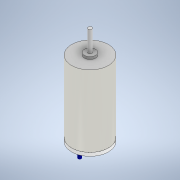
# Autodesk Inventor part: motor_noname
Saved by Autodesk Inventor 2021 (Build 250183000, 183)
## iProperties
Created: 2022-02-27
Part Number: motor_noname
Material: Generic
Document SubType Name: Modeling
Designer: ermoz
Density: 1 g/cm^3
Appearance: Default
Author: ermoz
Autodesk Inventor part; units mm, degrees
ref_plane "YZ Plane" through (0, 0, 0) normal (1, 0, 0) x (0, 1, 0)
ref_plane "XZ Plane" through (0, 0, 0) normal (0, 1, 0) x (-1, 0, 0)
ref_plane "XY Plane" through (0, 0, 0) normal (0, 0, 1) x (1, 0, 0)
sketch "Sketch1" plane through (0, 0, 0) normal (0, 1, 0) x (-1, 0, 0)
  circle A0 centre (0, 0) radius 4
  dimension "d0" = 8
  constraints: 1 centre point, 1 coincident
  measures "d0" diameter of A0
extrude "Extrusion1" add sketch "Sketch1" along normal blind 15.6
sketch "Sketch2" plane through (0, 15.6, 0) normal (0, 1, 0) x (1, 0, 0)
  circle A0 centre (0, 0) radius 4 projected
  circle A1 centre (0, 0) radius 1.2
  dimension "d3" = 2.4
  constraints: 1 centre point, 1 coincident
  measures "d3" diameter of A1
extrude "Extrusion2" add sketch "Sketch2" along normal blind 0.5 contours A1
sketch "Sketch3" plane through (0, 0, 0) normal (0, -1, 0) x (1, 0, 0)
  circle A0 centre (0, 0) radius 1.2 projected
  circle A1 centre (0, 0) radius 4
  constraints: 1 centre point, 1 coincident
extrude "Extrusion3" add sketch "Sketch3" along normal blind 0.75 separate body contours A0 | A1
sketch "Sketch4" plane through (0, 16.1, 0) normal (0, 1, 0) x (1, 0, 0)
  circle A0 centre (0, 0) radius 0.4
  dimension "d8" = 0.8
  constraints: 1 centre point, 1 coincident
  measures "d8" diameter of A0
extrude "Extrusion4" add sketch "Sketch4" along normal blind 4.6 separate body
sketch "Sketch5" plane through (0, -0.75, 0) normal (0, -1, 0) x (1, 0, 0)
  circle A0 centre (0, 2.25) radius 0.35
  circle A1 centre (0, -2.25) radius 0.35
  line L0 (0, 0) -> (2.0359, 0)
  dimension "d11" = 0.7
  dimension "d12" = 0.7
  dimension "d13" = 4.5
  constraints: 2 centre point, 2 end point, 1 horizontal, 1 symmetric about line
  measures "d11" diameter of A0
  measures "d12" diameter of A1
  measures "d13" distance of A0.centre A1.centre
extrude "Extrusion5" add sketch "Sketch5" along normal blind 2 separate body contours A1
extrude "Extrusion6" add sketch "Sketch5" along normal blind 2 separate body contours A0
body "Solid1"
body "Solid2"
body "Solid3"
body "Solid4"
body "Solid5"
